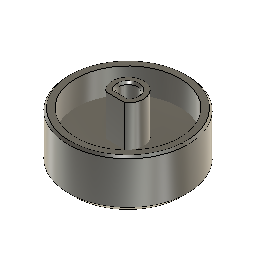
TOASTERknob (Autodesk Fusion 360 design; units mm, degrees)
Autodesk Fusion 360 part; units mm, degrees
note: some values were not read from the file. Set by a fixed rule: which sketch regions a step uses.
sketch "Sketch1" plane through (0, 0, 0) normal (0, 0, 1) x (1, 0, 0)
  circle A0 centre (0, 0) radius 19
  circle A1 centre (0, 0) radius 3
  line L0 (-2.2361, 0) -> (-2.2361, -2) construction
  line L1 (-2.2361, -2) -> (2.2361, -2)
  line L2 (2.2361, -2) -> (2.2361, 0) construction
  line L3 (2.2361, 0) -> (-2.2361, 0) construction
  line L4 (-0.75, -9) -> (-0.75, -15)
  arc A2 (-0.75, -15) -> (0.75, -15) centre (0, -15) ccw
  line L5 (0.75, -15) -> (0.75, -9)
  arc A3 (0.75, -9) -> (-0.75, -9) centre (0, -9) ccw
  line L6 (0, -8.25) -> (0, -15.75) construction
  line L7 (0, 1.75) -> (0, 22.5)
  dimension "d1" = 38
  dimension "d2" = 6
  dimension "d14" = 1.5
  dimension "d15" = 15
  dimension "d16" = 9
  dimension "d21" = 2
  constraint coincident A0.centre A1.centre
  constraint perpendicular L0 L1
  constraint parallel L0 L2
  constraint parallel L1 L3
  constraint coincident A1 L0.end
  constraint vertical L0
  constraint coincident A1 L1.end
  constraint coincident A0.centre L3
  constraint tangent L4 A2
  constraint tangent A2 L5
  constraint parallel L4 L5
  constraint tangent L5 A3
  constraint tangent L4 A3
  constraint midpoint A3 L6.start
  constraint midpoint A2 L6.end
  constraint vertical L6
  constraint collinear L6 L7
  measures "d1" diameter of A0
  measures "d2" diameter of A1
  measures "d14" diameter of A2
  measures "d15" distance of A0.centre A2.centre
  measures "d16" distance of A0.centre A3.centre
  measures "d21" distance of A0.centre L1
extrude "Extrude1" add sketch "Sketch1" along normal blind 16 thin wall 2.5 inside contours A0 | A1 L1 | A1 L1 | L4 A2 L5 A3
extrude "Extrude2" add sketch "Sketch1" along normal blind 8 contours A0 | A1 L1 | A1 L1 | L4 A2 L5 A3
extrude "Extrude3" add sketch "Sketch1" along normal blind 13 from surface at 8 thin wall 2 outside contours A1 L1 picked at (0.8282, -0.3221)
extrude "Extrude4" cut sketch "Sketch1" along normal blind 0.2 contours L4 A2 L5 A3
chamfer "Chamfer1" distance 2 angle 45 1 edges at (-17.7142, -6.8707, 0)
chamfer "Chamfer1" distance 0.2 angle 45 4 edges at (-0.75, -12, 0) (0, -15.75, 0) (0.75, -12, 0) (0, -8.25, 0)
chamfer "Chamfer1" distance 0.6 angle 45 3 edges at (0, 3, 21) (0, -2, 21) (-17.7142, -6.8707, 16)
